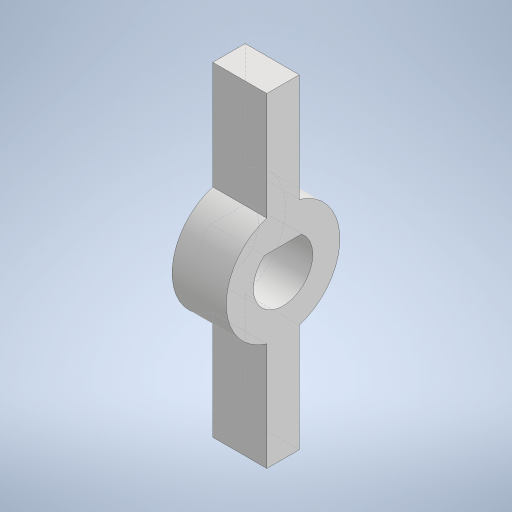
# Autodesk Inventor part: dshaft_fit_test
Saved by Autodesk Inventor 2023 (Build 270158000, 158)
## iProperties
Created: 2022-10-01
Part Number: dshaft_fit_test
Material: Generic
Document SubType Name: Modeling
Designer: carso
Density: 1 g/cm^3
Appearance: Default
Author: carso
Autodesk Inventor part; units mm, degrees
ref_plane "YZ Plane" through (0, 0, 0) normal (1, 0, 0) x (0, 1, 0)
ref_plane "XZ Plane" through (0, 0, 0) normal (0, 1, 0) x (-1, 0, 0)
ref_plane "XY Plane" through (0, 0, 0) normal (0, 0, 1) x (1, 0, 0)
sketch "Sketch1" plane through (0, 0, 0) normal (1, 0, 0) x (0, 1, 0)
  circle A0 centre (0, 0) radius 2.75
  line L0 (-2.75, 0) -> (2.15, 0)
  line L1 (2.15, 0) -> (2.15, -1.7146)
  line L2 (2.15, 0) -> (2.15, 1.7146)
  circle A1 centre (0, 0) radius 5.25
  line L3 (15, 1.5) -> (-15, 1.5)
  line L4 (-15, 1.5) -> (-15, -1.5)
  line L5 (-15, -1.5) -> (15, -1.5)
  line L6 (15, -1.5) -> (15, 1.5)
  line L7 (15, 1.5) -> (-15, -1.5) construction
  line L8 (-15, 1.5) -> (15, -1.5) construction
  point P0 (5.0312, 1.5)
  point P1 (-5.0312, 1.5)
  point P2 (-5.0312, -1.5)
  point P3 (5.0312, -1.5)
  dimension "d0" = 5.5
  dimension "d3" = 4.9
  dimension "d4" = 2.5
  dimension "d5" = 30
  dimension "d6" = 3
  constraints: 18 end point, 3 point on circle, 2 centre point, 2 coincident, 2 horizontal, 2 midpoint, 2 parallel, 2 perpendicular, 1 point on line
  measures "d0" diameter of A0
  measures "d3" distance of L0.start L0.end
  measures "d4" radial gap between concentric circles of A1 A0
  measures "d5" distance of L5.end L4.end
  measures "d6" distance between parallel lines of L5 L3
extrude "Extrusion1" add sketch "Sketch1" along normal blind 5 contours A0 L5 L1 L2 L3 | A0 L3 A1 L5 | L3 L2 A0 | A0 L3 A1 | L5 A1 A0 | A0 L1 L5 | L3 L6 L5 A1 | A0 L5 A1 L3 | A1 L5 L4 L3 picked at (2.168, 1.6198) picked at (2.168, -1.6198)
body "Solid1"
